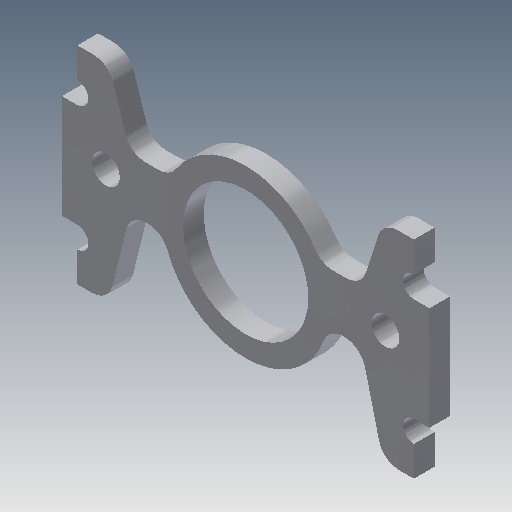
# Autodesk Inventor part: 足首_サブフレーム_1_2
Saved by Autodesk Inventor 2017.3 (Build 213256000, 256)
## iProperties
Created: 2016-04-30
Part Number: 足首_サブフレーム_1_2
Material: アルミニウム 2014-T4
Document SubType Name: Modeling
Designer: hiroaki
Density: 2.8 g/cm^3
Appearance: サテン
Mass: 1.85247 g
Surface Area: 10.2984 cm^2
Volume: 0.661596 cm^3
Author: hiroaki
Autodesk Inventor part; units mm, degrees
ref_plane "YZ Plane" through (0, 0, 0) normal (1, 0, 0) x (0, 1, 0)
ref_plane "XZ Plane" through (0, 0, 0) normal (0, 1, 0) x (-1, 0, 0)
ref_plane "XY Plane" through (0, 0, 0) normal (0, 0, 1) x (1, 0, 0)
sketch "スケッチ1" plane through (0, 0, 0) normal (0, 0, 1) x (1, 0, 0)
  circle A0 centre (0, 0) radius 10.5 construction
  circle A1 centre (-13.5, 1) radius 1.35
  line L0 (-13.5, 28) -> (13.5, 28) construction
  line L1 (13.5, 28) -> (13.5, 1) construction
  line L2 (13.5, 1) -> (-13.5, 1) construction
  line L3 (-13.5, 1) -> (-13.5, 28) construction
  circle A2 centre (-13.5, 28) radius 1.35
  circle A3 centre (13.5, 1) radius 1.35
  circle A4 centre (13.5, 28) radius 1.35
  line L4 (-16.25, 10) -> (-16.25, 7.1)
  line L5 (-16.25, 10) -> (16.25, 10)
  line L6 (16.25, 10) -> (16.25, 7.1)
  line L7 (-16.25, -7.1) -> (-16.25, -10)
  line L8 (-16.25, -10) -> (16.25, -10)
  line L9 (16.25, -7.1) -> (16.25, -10)
  line L10 (-16.25, 5) -> (-17.75, 5)
  line L11 (-17.75, 5) -> (-17.75, -5)
  line L12 (-17.75, -5) -> (-16.25, -5)
  arc A5 (-16.25, 5) -> (-16.25, 7.1) centre (-16.25, 6.05) ccw
  arc A6 (-16.25, -7.1) -> (-16.25, -5) centre (-16.25, -6.05) ccw
  line L13 (16.25, 5) -> (17.75, 5)
  line L14 (17.75, 5) -> (17.75, -5)
  line L15 (17.75, -5) -> (16.25, -5)
  arc A7 (16.25, 7.1) -> (16.25, 5) centre (16.25, 6.05) ccw
  line L16 (0, 28) -> (0, 0) construction
  arc A8 (16.25, -5) -> (16.25, -7.1) centre (16.25, -6.05) ccw
  line L17 (-17.75, 0) -> (17.75, 0) construction
  circle A9 centre (0, 0) radius 6.05
  point P0 (0, 10)
  dimension "d8" = 21
  dimension "d10" = 27
  dimension "d12" = 1
  dimension "d13" = 2.7
  dimension "d38" = 27
  dimension "d44" = 27
  dimension "d47" = 1.05
  dimension "d48" = 32.5
  dimension "d49" = 1.5
  dimension "d50" = 10
  dimension "d51" = 5
  dimension "d52" = 12.1
  dimension "d64" = 1.5
  constraints: 36 end point, 10 centre point, 9 perpendicular, 8 point on circle, 7 vertical alignment, 5 midpoint, 5 vertical, 4 horizontal, 4 tangent, 3 coincident, 3 equal radius, 2 parallel, 2 symmetric about line, 1 horizontal alignment, 7 other
  measures "d8" diameter of A0
  measures "d10" distance of L0.start L0.end
  measures "d12" distance from line of point (0, 0) L2
  measures "d13" diameter of A1
  measures "d38" distance of A1.centre A2.centre
  measures "d44" distance of A1.centre A3.centre
  measures "d47" radius of A5
  measures "d48" distance of L4.start L5.end
  measures "d49" distance between parallel lines of L11 L4
  measures "d50" distance between parallel lines of L12 L10
  measures "d51" distance between parallel lines of L5 L10
  measures "d52" diameter of A9
  measures "d64" distance of L14.end L15.end
extrude "押し出し1" add sketch "スケッチ1" along normal blind 2 contours L5 L6 A7 L13 L14 L15 A8 L9 L8 L7 A6 L12 L11 L10 A5 L4
sketch "スケッチ3" plane through (0, 0, 2) normal (0, 0, 1) x (1, 0, 0)
  circle A0 centre (0, 0) radius 6.05 projected
  circle A1 centre (13.5, 1) radius 1.35 projected
  circle A2 centre (-13.5, 1) radius 1.35 projected
  line L0 (16.25, 10) -> (-16.25, 10) projected
  line L1 (-11.154, 3.5) -> (-7.2493, 3.5)
  line L2 (-11.154, -1.5) -> (-7.909, -1.5)
  line L3 (-13.5, 1) -> (13.5, 1) construction
  arc A3 (7.2493, 3.5) -> (-7.2493, 3.5) centre (0, 0) ccw
  line L4 (7.2493, 3.5) -> (11.154, 3.5)
  line L5 (-14.3875, 13.5275) -> (14.3875, 13.5275)
  line L6 (0, 0) -> (0, 10) construction
  arc A4 (-7.909, -1.5) -> (7.909, -1.5) centre (0, 0) ccw
  line L7 (7.909, -1.5) -> (11.154, -1.5)
  line L8 (14.3875, -14.6128) -> (-14.3875, -14.6128)
  line L9 (-16.25, -10) -> (16.25, -10) projected
  line L10 (-14.3875, -14.6128) -> (-11.154, -1.5)
  line L11 (-11.154, 3.5) -> (-14.3875, 13.5275)
  circle A5 centre (-13.5, 1) radius 3 construction
  line L12 (11.154, -1.5) -> (14.3875, -14.6128)
  line L13 (11.154, 3.5) -> (14.3875, 13.5275)
  line L14 (-13.25, 10) -> (-16.25, 10) construction
  line L15 (-13.25, -10) -> (-16.25, -10) construction
  line L16 (13.25, 10) -> (16.25, 10) construction
  line L17 (16.25, -10) -> (13.25, -10) construction
  dimension "d68" = 2.5
  dimension "d69" = 2
  dimension "d73" = 6
  dimension "d74" = 3
  constraints: 32 end point, 8 point on line, 7 horizontal, 4 coincident, 4 point on circle, 4 symmetric about line, 3 centre point, 3 collinear, 3 vertical alignment, 2 horizontal alignment, 1 concentric, 1 midpoint, 1 tangent, 1 other
  measures "d68" distance between parallel lines of L1 L3
  measures "d69" radial gap between concentric circles of A3 A0
  measures "d73" diameter of A5
  measures "d74" distance of L14.start L0.end
extrude "押し出し3" cut sketch "スケッチ3" against normal blind 10 contours L13 L4 A3 L1 L11 L0 | L2 A4 L7 L12 L9 L10
fillet "フィレット2" radius 2 12 edges at (-11.154, 3.5, 1) (-7.2493, 3.5, 1) (7.909, -1.5, 1) (7.2493, 3.5, 1) (11.154, 3.5, 1) (-7.909, -1.5, 1) (-11.154, -1.5, 1) (11.154, -1.5, 1) (-13.25, -10, 1) (-13.25, 10, 1) (13.25, -10, 1) (13.25, 10, 1)
equation "\"d38\" = d10"
equation "\"d44\" = d10"
equation "\"d50\" = d11"
equation "\"d51\" = d28"
equation "\"d64\" = d49"
equation "\"d11\" = 10"
equation "\"d28\" = 5"
